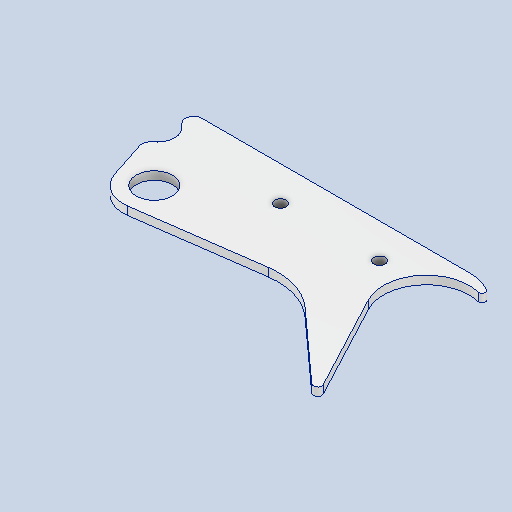
# Autodesk Inventor part: hook-top-plate
Saved by Autodesk Inventor 2025.2 (Build 292293000, 293)
## iProperties
Created: 2025-03-18
Part Number: hook-top-plate
Material: Aluminum 6061
Document SubType Name: Sheet Metal
Designer: mathe
Density: 2.7 g/cm^3
Sheet Metal Rule: Default
Appearance: Aluminum - Flat
Author: mathe
Autodesk Inventor part; units mm, degrees
ref_plane "YZ Plane" through (0, 0, 0) normal (1, 0, 0) x (0, 1, 0)
ref_plane "XZ Plane" through (0, 0, 0) normal (0, 1, 0) x (-1, 0, 0)
ref_plane "XY Plane" through (0, 0, 0) normal (0, 0, 1) x (1, 0, 0)
sketch "Sketch1" plane through (0, 0, 0) normal (0, 1, 0) x (-1, 0, 0)
  line L0 (103.4591, 16.4441) -> (104.7625, 17.6511)
  arc A0 (104.7625, 17.6511) -> (105.6235, 20.966) centre (102.6053, 19.9807) ccw
  line L1 (105.6235, 20.966) -> (100.9494, 35.2839)
  arc A1 (100.9494, 35.2839) -> (87.8224, 43.4902) centre (89.4801, 31.5396) ccw
  line L2 (87.8224, 43.4902) -> (40.332, 36.9027)
  arc A2 (19.8124, 43.2164) -> (40.332, 36.9027) centre (36.8421, 62.0618) ccw
  line L3 (19.8124, 43.2164) -> (-6.8947, 67.3504)
  arc A3 (-6.8947, 67.3504) -> (-9.362, 65.4298) centre (-7.959, 66.1726) ccw
  line L4 (-9.362, 65.4298) -> (10.1942, 28.4903)
  arc A4 (-8.303, 4.7241) -> (10.1942, 28.4903) centre (-4.3971, 20.7654) ccw
  arc A5 (-8.303, 4.7241) -> (-9.218, 2.3787) centre (-8.6034, 3.4901) ccw
  arc A6 (-9.218, 2.3787) -> (0, 0) centre (0, 19.05) ccw
  line L5 (0, 0) -> (102.7651, 0)
  arc A7 (102.7651, 0) -> (105.0946, 5.3323) centre (102.7651, 3.175) ccw
  line L6 (105.0946, 5.3323) -> (103.1146, 7.4705)
  arc A8 (103.4591, 16.4441) -> (103.1146, 7.4705) centre (107.7737, 11.785) ccw
  circle A9 centre (89.4801, 31.5396) radius 6.985
  circle A10 centre (21.1327, 13.2882) radius 2.2479
  circle A11 centre (59.2327, 13.2882) radius 2.2479
  point P0 (0, 0)
  point P1 (-8.303, 4.7241)
  point P2 (-9.218, 2.3787)
  point P3 (0, 0)
  point P4 (102.7651, 0)
  point P5 (105.0946, 5.3323)
  point P6 (105.6235, 20.966)
  point P7 (19.8124, 43.2164)
  point P8 (-9.362, 65.4298)
  point P9 (10.1942, 28.4903)
extrude "Plate1" add sketch "Sketch1" along normal blind 3.175
equation "\"d0\" = Thickness"
equation "\"BendRadius\" = Thickness"
equation "\"BendReliefWidth\" = Thickness"
equation "\"BendReliefDepth\" = 0.5 * Thickness"
equation "\"CornerReliefSize\" = 4 * Thickness"
equation "\"MinimumRemnant\" = 2 * Thickness"
equation "\"TransitionRadius\" = BendRadius"
equation "\"JacobiRadiusSize\" = BendRadius"
equation "\"GapSize\" = Thickness"
equation "\"Thickness\" = 3.175"
body "Solid1"
